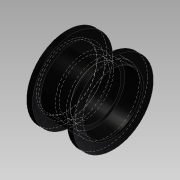
# Autodesk Inventor part: V-Slot Idler Pulley
Saved by Autodesk Inventor 2015 (Build 190159000, 159)
## iProperties
Created: 2013-06-20
Part Number: V-Slot Idler Pulley
Material: Acetal Resin, Black
Document SubType Name: Modeling
Designer: Jon Hollander
Density: 1.425 g/cm^3
Mass: 1.57207 g
Surface Area: 20.7951 cm^2
Volume: 1.1032 cm^3
Appearance: Smooth - Black
Author: Jon Hollander
Autodesk Inventor part; units mm, degrees
ref_plane "YZ Plane" through (0, 0, 0) normal (1, 0, 0) x (0, 1, 0)
ref_plane "XZ Plane" through (0, 0, 0) normal (0, 1, 0) x (-1, 0, 0)
ref_plane "XY Plane" through (0, 0, 0) normal (0, 0, 1) x (1, 0, 0)
sketch "Sketch1" plane through (0, 0, 0) normal (0, 0, 1) x (1, 0, 0)
  line L0 (0, 0) -> (5, 0)
  line L1 (0, 0) -> (0, 15.689) construction
  line L2 (0, 6.945) -> (1.55, 6.945)
  line L3 (1.55, 6.945) -> (1.55, 7.987)
  line L4 (1.55, 7.987) -> (6.05, 7.987)
  line L5 (6.35, 8.287) -> (6.35, 11)
  line L6 (6.35, 11) -> (4.75, 11)
  line L7 (4.75, 11) -> (4.75, 8.75)
  line L8 (4.75, 8.75) -> (0, 8.75)
  line L9 (6.35, 8.287) -> (6.05, 7.987)
  line L10 (0, 6.945) -> (-1.55, 6.945)
  line L11 (-1.55, 6.945) -> (-1.55, 7.987)
  line L12 (-1.55, 7.987) -> (-6.05, 7.987)
  line L13 (-6.35, 8.287) -> (-6.35, 11)
  line L14 (-6.35, 11) -> (-4.75, 11)
  line L15 (-4.75, 11) -> (-4.75, 8.75)
  line L16 (-4.75, 8.75) -> (0, 8.75)
  line L17 (-6.35, 8.287) -> (-6.05, 7.987)
  point P0 (6.35, 7.987)
  point P1 (-6.35, 7.987)
  dimension "d0" = 5
  dimension "d1" = 1.55
  dimension "d2" = 13.89
  dimension "d3" = 15.974
  dimension "d5" = 22
  dimension "d6" = 17.5
  dimension "d7" = 1.6
  dimension "d8" = 4.75
  dimension "d9" = 0.3
  dimension "d10" = 0.3
  constraints: 36 end point, 8 symmetric about line, 6 point on line, 4 parallel, 4 perpendicular, 1 horizontal
  measures "d0" distance of L0.start L0.end
  measures "d1" distance of L2.start L2.end
  measures "d2" diameter of L2 L0
  measures "d3" diameter of L4 L0
  measures "d5" diameter of L6 L0
  measures "d6" diameter of L8 L0
  measures "d7" distance of L5.end L6.end
  measures "d8" distance between parallel lines of L1 L7
  measures "d9" distance of L5.start point (6.35, 7.987)
  measures "d10" distance of L4.end point (6.35, 7.987)
revolve "Revolution1" add sketch "Sketch1" angle 360 about axis through (0, 0, 0) along (1, 0, 0)
equation "\"d10\" = d9"
body "Solid1"
